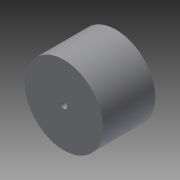
# Autodesk Inventor part: tendeur_roue
Saved by Autodesk Inventor 2015 (Build 190159000, 159)
## iProperties
Created: 2015-09-12
Part Number: tendeur_roue
Material: Générique
Document SubType Name: Modeling
Designer: astralien3000
Density: 1 g/cm^3
Appearance: Par défaut
Author: astralien3000
Autodesk Inventor part; units mm, degrees
ref_plane "YZ Plane" through (0, 0, 0) normal (1, 0, 0) x (0, 1, 0)
ref_plane "XZ Plane" through (0, 0, 0) normal (0, 1, 0) x (-1, 0, 0)
ref_plane "XY Plane" through (0, 0, 0) normal (0, 0, 1) x (1, 0, 0)
sketch "Esquisse1" plane through (0, 0, 0) normal (0, 1, 0) x (-1, 0, 0)
  circle A0 centre (0, 0) radius 0.5
  circle A1 centre (0, 0) radius 6
  dimension "d0" = 12
  dimension "d1" = 1
  constraints: 2 centre point, 2 coincident
  measures "d0" diameter of A1
  measures "d1" diameter of A0
extrude "Extrusion1" add sketch "Esquisse1" along normal blind 8
